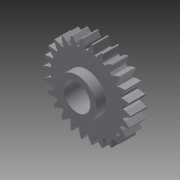
# Autodesk Inventor part: Part3
Saved by Autodesk Inventor 2015 SP1 (Build 190203100, 203)
## iProperties
Created: 2015-06-02
Part Number: Part3
Material: Generic
Document SubType Name: Modeling
Designer: pltwe4
Density: 1 g/cm^3
Appearance: Default
Author: pltwe4
Autodesk Inventor part; units mm, degrees
ref_plane "YZ Plane" through (0, 0, 0) normal (1, 0, 0) x (0, 1, 0)
ref_plane "XZ Plane" through (0, 0, 0) normal (0, 1, 0) x (-1, 0, 0)
ref_plane "XY Plane" through (0, 0, 0) normal (0, 0, 1) x (1, 0, 0)
sketch "Sketch1" plane through (0, 0, 0) normal (0, 1, 0) x (-1, 0, 0)
  circle A0 centre (0, 0) radius 13.5
  line L0 (11.1312, 1) -> (11.9696, 0.875)
  line L1 (11.9696, 0.875) -> (13.4987, 0.1875)
  line L2 (13.4987, -0.1875) -> (11.9696, -0.875)
  line L3 (11.9696, -0.875) -> (11.1312, -1)
  line L4 (-18.9, 0) -> (18.9, 0) projected
  circle A1 centre (0, 0) radius 12.0015 construction
  circle A2 centre (0, 0) radius 11.176
  dimension "d2" = 24.003
  dimension "d0" = 27
  dimension "d3" = 2
  dimension "d4" = 0.375
  dimension "d5" = 1.75
  dimension "d8" = 22.352
  constraints: 8 end point, 4 point on circle, 3 coincident, 2 centre point, 5 other
  measures "d0" diameter of A0
  measures "d3" distance of L0.start L3.end
  measures "d4" distance of L1.end L2.start
  measures "d5" distance of L0.end L2.end
  measures "d8" diameter of A2
extrude "Extrusion1" add sketch "Sketch1" along normal blind 5 contours A2 L4 | L4 A2
extrude "Extrusion2" add sketch "Sketch1" along normal blind 5 contours L4 A2 L0 L1 A0 | A0 L2 L3 A2 L4 picked at (12.2152, 0.2917) picked at (12.2152, -0.2917)
pattern_circular "Circular Pattern1" count 26 over 360 about axis through (0, 0, 0) along (0, 1, 0) of "Extrusion2"
sketch "Sketch2" plane through (0, 0, 0) normal (0, -1, 0) x (1, 0, 0)
  circle A0 centre (0, 0) radius 4.0625
  dimension "d14" = 8.125
  constraints: 1 centre point, 1 coincident
  measures "d14" diameter of A0
extrude "Extrusion3" cut sketch "Sketch2" against normal blind 5
sketch "Sketch3" plane through (0, 0, 0) normal (0, -1, 0) x (1, 0, 0)
  circle A0 centre (0, 0) radius 6
  circle A1 centre (0, 0) radius 4.0625 projected
  dimension "d17" = 12
  constraints: 1 centre point, 1 coincident
  measures "d17" diameter of A0
extrude "Extrusion4" add sketch "Sketch3" along normal blind 3
body "Solid1"
